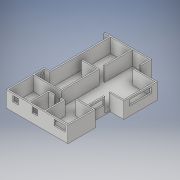
# Autodesk Inventor part: Haus
Saved by Autodesk Inventor 2019 (Build 230136000, 136)
## iProperties
Created: 2019-04-30
Part Number: Haus
Material: Generisch
Document SubType Name: Modeling
Designer: niede
Density: 1 g/cm^3
Appearance: Vorgabe
Author: niede
Autodesk Inventor part; units mm, degrees
ref_plane "YZ Plane" through (0, 0, 0) normal (1, 0, 0) x (0, 1, 0)
ref_plane "XZ Plane" through (0, 0, 0) normal (0, 1, 0) x (-1, 0, 0)
ref_plane "XY Plane" through (0, 0, 0) normal (0, 0, 1) x (1, 0, 0)
sketch "Skizze2" plane through (0, 0, 0) normal (0, 1, 0) x (-1, 0, 0)
  line L0 (0, 0) -> (11230, 0)
  line L1 (11230, 0) -> (11230, -6920)
  line L2 (11230, -6920) -> (10230, -6920)
  line L3 (10230, -6920) -> (10230, -17740)
  line L4 (10230, -17740) -> (11230, -17740)
  line L5 (11230, -17740) -> (11230, -17980)
  line L6 (11230, -17980) -> (2740, -17980)
  line L7 (2740, -17980) -> (2740, -14980)
  line L8 (2740, -14980) -> (-1250, -14980)
  line L9 (-1250, -14980) -> (-1250, -8870)
  line L10 (-1250, -8870) -> (1180, -8870)
  line L11 (1180, -8870) -> (1180, -4980)
  line L12 (1180, -4980) -> (0, -4980)
  line L13 (0, -4980) -> (0, 0)
  dimension "d6" = 11230
  dimension "d7" = 6920
  dimension "d8" = 1000
  dimension "d9" = 10820
  dimension "d10" = 240
  dimension "d11" = 8490
  dimension "d12" = 3000
  dimension "d13" = 3990
  dimension "d14" = 6110
  dimension "d15" = 2430
  dimension "d16" = 3890
  dimension "d17" = 1180
  constraints: 28 end point, 9 perpendicular, 2 point on line, 2 vertical, 1 horizontal
  measures "d6" distance of L0.start L0.end
  measures "d7" distance of L0.end L1.end
  measures "d8" distance of L1.end L2.end
  measures "d9" distance of L2.end L3.end
  measures "d10" distance of L4.end L5.end
  measures "d11" distance of L5.end L6.end
  measures "d12" distance of L6.end L7.end
  measures "d13" distance of L7.end L8.end
  measures "d14" distance of L8.end L9.end
  measures "d15" distance of L9.end L10.end
  measures "d16" distance of L10.end L11.end
  measures "d17" distance of L11.end L12.end
extrude "Fundament" add sketch "Skizze2" along normal blind 300
sketch "Skizze3" plane through (0, 300, 0) normal (0, 1, 0) x (1, 0, 0)
  line L0 (-11230, 0) -> (0, 0) projected
  line L1 (0, 0) -> (0, 4980) projected
  line L2 (0, 4980) -> (-1180, 4980) projected
  line L3 (-1180, 4980) -> (-1180, 8870) projected
  line L4 (-1180, 8870) -> (1250, 8870) projected
  line L5 (1250, 8870) -> (1250, 14980) projected
  line L6 (1250, 14980) -> (-2740, 14980) projected
  line L7 (-2740, 14980) -> (-2740, 17980) projected
  line L8 (-2740, 17980) -> (-11230, 17980) projected
  line L9 (-10230, 17740) -> (-10230, 6920) projected
  line L10 (-10230, 6920) -> (-11230, 6920) projected
  line L11 (-11230, 6920) -> (-11230, 0) projected
  line L12 (-11230, 0) -> (-11230, 6920) projected
  line L13 (-11230, 0) -> (-11230, 6920)
  line L14 (-11230, 6920) -> (-10230, 6920)
  line L15 (-10230, 17740) -> (-11230, 17740) projected
  line L16 (-10230, 17740) -> (-11230, 17740)
  line L17 (-11230, 17980) -> (-2740, 17980) projected
  line L18 (-11230, 17740) -> (-11230, 17980)
  line L19 (-11230, 17980) -> (-2740, 17980)
  line L20 (-2740, 17980) -> (-2740, 15980)
  line L21 (1250, 14980) -> (1250, 8870)
  line L22 (-1180, 7870) -> (-1180, 4980)
  line L23 (0, 4980) -> (0, 0)
  line L24 (0, 0) -> (-11230, 0)
  line L25 (-10990, 240) -> (-240, 240)
  line L26 (-240, 240) -> (-240, 4740)
  line L27 (-240, 4740) -> (-1420, 4740)
  line L28 (-1420, 4740) -> (-1420, 7870)
  line L29 (-1420, 7870) -> (-1180, 7870)
  line L30 (-10990, 240) -> (-10990, 6680)
  line L31 (-5990, 6680) -> (-5990, 11680)
  line L32 (-5990, 11680) -> (-8990, 11680)
  line L33 (-8990, 11680) -> (-8990, 11440)
  line L34 (-8990, 11440) -> (-6230, 11440)
  line L35 (-6230, 11440) -> (-6230, 6920)
  line L36 (-9990, 6920) -> (-9990, 17740)
  line L37 (-9990, 17740) -> (-6230, 17740)
  line L38 (-6230, 17740) -> (-6230, 12680)
  line L39 (-6230, 12680) -> (-5990, 12680)
  line L40 (-5990, 12680) -> (-5990, 17740)
  line L41 (-5990, 17740) -> (-2980, 17740)
  line L42 (-2980, 14740) -> (1010, 14740)
  line L43 (1010, 14740) -> (1010, 9110)
  line L44 (1010, 9110) -> (-1420, 9110)
  line L45 (-1420, 9110) -> (-1420, 8870)
  line L46 (-1420, 8870) -> (-952.7911, 8870)
  line L47 (-1420, 4740) -> (-3420, 4740)
  line L48 (-3420, 4740) -> (-3420, 4980)
  line L49 (-3420, 4980) -> (-1420, 4980)
  line L50 (-10990, 4740) -> (-6230, 4740)
  line L51 (-6230, 4740) -> (-5990, 4740)
  line L52 (-5990, 4740) -> (-5990, 6680)
  line L53 (-10990, 4980) -> (-6230, 4980)
  line L54 (-6230, 4980) -> (-6230, 6920)
  line L55 (-6990, 240) -> (-6990, 3500)
  line L56 (-6990, 3500) -> (-5990, 3500)
  line L57 (-5990, 3500) -> (-5990, 3740)
  line L58 (-5990, 3740) -> (-7230, 3740)
  line L59 (-7230, 3740) -> (-7230, 240)
  line L60 (-4480, 240) -> (-4480, 3500)
  line L61 (-4480, 3500) -> (-4990, 3500)
  line L62 (-4990, 3500) -> (-4990, 3740)
  line L63 (-4990, 3740) -> (-4240, 3740)
  line L64 (-4240, 3740) -> (-4240, 240)
  line L65 (-10990, 6680) -> (-9990, 6680)
  line L66 (-9990, 6680) -> (-9990, 6920)
  line L67 (-2740, 14980) -> (-2980, 14980)
  line L68 (-2740, 15980) -> (-2980, 15980)
  line L69 (-2980, 17740) -> (-2980, 15980)
  line L70 (-2980, 14980) -> (-2980, 14740)
  dimension "d20" = 5000
  dimension "d21" = 240
  dimension "d23" = 240
  dimension "d24" = 240
  dimension "d25" = 240
  dimension "d26" = 240
  dimension "d27" = 1000
  dimension "d28" = 240
  dimension "d29" = 240
  dimension "d30" = 240
  dimension "d31" = 240
  dimension "d33" = 240
  dimension "d34" = 240
  dimension "d35" = 240
  dimension "d36" = 240
  dimension "d37" = 240
  dimension "d38" = 240
  dimension "d39" = 1000
  dimension "d40" = 1000
  dimension "d41" = 5000
  dimension "d54" = 1000
  dimension "d55" = 2000
  dimension "d56" = 240
  dimension "d57" = 240
  dimension "d58" = 240
  dimension "d59" = 240
  dimension "d60" = 3760
  dimension "d61" = 2510
  dimension "d62" = 1000
  dimension "d63" = 1000
  dimension "d64" = 240
  dimension "d65" = 240
  dimension "d66" = 90
  dimension "d67" = 2300
  dimension "d68" = 10000
  dimension "d69" = 2202.7911
  dimension "d70" = 7480
  dimension "d107" = 240
  dimension "d108" = 1000
  dimension "d109" = 240
  constraints: 112 end point, 34 perpendicular, 17 point on line, 5 collinear, 5 parallel, 4 vertical, 2 horizontal
  measures "d20" distance of L30.end L31.start
  measures "d21" distance between parallel lines of L0 L25
  measures "d23" distance between parallel lines of L11 L30
  measures "d24" distance between parallel lines of L1 L26
  measures "d25" distance between parallel lines of L2 L27
  measures "d26" distance between parallel lines of L3 L28
  measures "d27" distance between parallel lines of L29 L46
  measures "d28" distance between parallel lines of L4 L44
  measures "d29" distance of L3.end L45.end
  measures "d30" distance between parallel lines of L5 L43
  measures "d31" distance between parallel lines of L6 L42
  measures "d33" distance between parallel lines of L8 L41
  measures "d34" distance between parallel lines of L40 L38
  measures "d35" distance between parallel lines of L8 L37
  measures "d36" distance between parallel lines of L9 L36
  measures "d37" distance of L32.end L33.end
  measures "d38" distance between parallel lines of L31 L35
  measures "d39" distance from line of L36 L33.end
  measures "d40" distance from line of L32 L39.end
  measures "d41" distance of L31.start L31.end
  measures "d54" distance between parallel lines of L47 L63
  measures "d55" distance of L48.end L49.end
  measures "d56" distance of L47.end L48.end
  measures "d57" distance between parallel lines of L64 L60
  measures "d58" distance between parallel lines of L55 L59
  measures "d59" distance between parallel lines of L58 L56
  measures "d60" distance between parallel lines of L30 L59
  measures "d61" distance between parallel lines of L55 L60
  measures "d62" distance of L61.end L56.end
  measures "d63" distance of L55.end L56.end
  measures "d64" distance between parallel lines of L53 L50
  measures "d65" distance between parallel lines of L10 L65
  measures "d66" angle of L49 L5
  measures "d67" distance between parallel lines of L6 L39
  measures "d68" distance between parallel lines of L6 L53
  measures "d69" distance from line of L46.end L5
  measures "d70" distance from line of L50.end L5
  measures "d107" distance between parallel lines of L70 L7
  measures "d108" distance between parallel lines of L67 L68
  measures "d109" distance between parallel lines of L7 L69
extrude "Wände" add sketch "Skizze3" along normal blind 2600 contours L11 L10 L9 L15 L18 L8 L7 L68 L69 L41 L40 L39 L38 L37 L36 L66 L65 L30 L25 L26 L27 L28 L29 L3 L2 L1 L0 | L46 L45 L44 L43 L42 L70 L67 L6 L5 L4 | L28 L47 L48 L49 | L25 L60 L61 L62 L63 L64 | L25 L59 L58 L57 L56 L55 | L30 L53 L54 L35 L34 L33 L32 L31 L52 L51 L50
sketch "Skizze6" plane through (-11230, 0, 0) normal (0, 0, 1) x (1, 0, 0)
  line L0 (11230, 0) -> (11230, 2900) projected
  line L1 (0, 2900) -> (11230, 2900) projected
  line L2 (1230, 2600) -> (2230, 2600)
  line L3 (2230, 2600) -> (2230, 1600)
  line L4 (2230, 1600) -> (1230, 1600)
  line L5 (1230, 1600) -> (1230, 2600)
  line L6 (4730, 2600) -> (5730, 2600)
  line L7 (5730, 2600) -> (5730, 1600)
  line L8 (5730, 1600) -> (4730, 1600)
  line L9 (4730, 1600) -> (4730, 2600)
  line L10 (8730, 2600) -> (10730, 2600)
  line L11 (10730, 2600) -> (10730, 1600)
  line L12 (10730, 1600) -> (8730, 1600)
  line L13 (8730, 1600) -> (8730, 2600)
  dimension "d75" = 1000
  dimension "d76" = 1000
  dimension "d77" = 2500
  dimension "d78" = 1000
  dimension "d79" = 2000
  dimension "d80" = 3000
  dimension "d81" = 300
  dimension "d84" = 500
  dimension "d99" = 300
  dimension "d100" = 1000
  constraints: 24 end point, 6 parallel, 3 horizontal, 3 perpendicular, 2 point on line
  measures "d75" distance of L4.end L2.start
  measures "d76" distance of L2.start L2.end
  measures "d77" distance between parallel lines of L9 L3
  measures "d78" distance of L6.start L6.end
  measures "d79" distance of L10.start L10.end
  measures "d80" distance between parallel lines of L7 L13
  measures "d81" distance between parallel lines of L1 L2
  measures "d84" distance between parallel lines of L0 L11
  measures "d99" distance between parallel lines of L1 L10
  measures "d100" distance between parallel lines of L10 L12
extrude "Fenster_West" cut sketch "Skizze6" against normal blind 240
sketch "Skizze8" plane through (1250, 0, -8870) normal (1, 0, 0) x (0, 0, -1)
  line L0 (0, 2900) -> (6110, 2900) projected
  line L1 (0, 0) -> (0, 2900) projected
  line L2 (1000, 2600) -> (5000, 2600)
  line L3 (5000, 2600) -> (5000, 1600)
  line L4 (5000, 1600) -> (1000, 1600)
  line L5 (1000, 1600) -> (1000, 2600)
  point P0 (-8870, 0)
  point P1 (0, 300)
  dimension "d87" = 300
  dimension "d88" = 4000
  dimension "d89" = 1000
  dimension "d90" = 1000
  constraints: 8 end point, 2 parallel, 1 horizontal, 1 perpendicular
  measures "d87" distance between parallel lines of L0 L2
  measures "d88" distance of L3.end L4.end
  measures "d89" distance between parallel lines of L1 L5
  measures "d90" distance of L2.end L3.end
extrude "Fenster_Süden_1" cut sketch "Skizze8" against normal blind 240
sketch "Skizze10" plane through (-1180, 0, -4980) normal (1, 0, 0) x (0, 0, -1)
  line L0 (2890, 300) -> (2890, 2900) projected
  line L1 (0, 2900) -> (2890, 2900) projected
  line L2 (0, 0) -> (0, 2900) projected
  line L3 (250, 2600) -> (2640, 2600)
  line L4 (2640, 2600) -> (2640, 1600)
  line L5 (2640, 1600) -> (250, 1600)
  line L6 (250, 1600) -> (250, 2600)
  point P0 (-4980, 0)
  dimension "d101" = 300
  dimension "d102" = 250
  dimension "d103" = 250
  dimension "d104" = 1000
  constraints: 8 end point, 2 parallel, 1 horizontal, 1 perpendicular
  measures "d101" distance between parallel lines of L1 L3
  measures "d102" distance between parallel lines of L2 L6
  measures "d103" distance between parallel lines of L0 L4
  measures "d104" distance between parallel lines of L3 L5
extrude "Fenster_Süden_2" cut sketch "Skizze10" against normal blind 240
sketch "Skizze9" plane through (-11230, 0, -6920) normal (-1, 0, 0) x (0, 0, 1)
  line L0 (0, 2900) -> (6920, 2900) projected
  line L1 (0, 0) -> (0, 2900) projected
  line L2 (450, 2600) -> (950, 2600)
  line L3 (950, 2600) -> (950, 2100)
  line L4 (950, 2100) -> (450, 2100)
  line L5 (450, 2100) -> (450, 2600)
  dimension "d93" = 300
  dimension "d94" = 450
  dimension "d95" = 500
  dimension "d96" = 500
  constraints: 8 end point, 2 parallel, 1 horizontal, 1 perpendicular
  measures "d93" distance between parallel lines of L0 L2
  measures "d94" distance between parallel lines of L1 L5
  measures "d95" distance of L3.end L4.end
  measures "d96" distance of L2.end L3.end
extrude "Fenster_Nord" cut sketch "Skizze9" against normal blind 240
